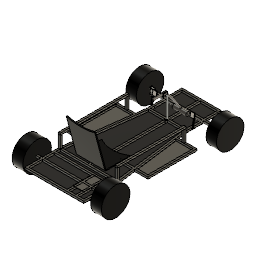
Go Kart Assembly.F3d (Autodesk Fusion 360 archive; units mm, degrees)
design "Go Kart Design"
Autodesk Fusion 360 part; units mm, degrees
note: some values were not read from the file. Chosen so that the rebuilt part matches the saved one: which bodies a step acts on; which face or edge a step refers to. Set by a fixed rule: which sketch regions a step uses.
(part 1 of 2)
sketch "Sketch1" plane through (0, 0, 0) normal (0, 0, 1) x (1, 0, 0)
  line L0 (139.7, 355.6) -> (279.4, 355.6)
  line L1 (279.4, 355.6) -> (279.4, 101.6)
  line L2 (279.4, 101.6) -> (139.7, 101.6)
  line L3 (139.7, 101.6) -> (139.7, 355.6)
  line L4 (139.7, 101.6) -> (160.7997, 101.6)
  line L5 (150.2738, 355.6) -> (139.7, 355.6)
  line L6 (139.7, 355.6) -> (139.7, 101.6)
  line L7 (239.1738, 355.6) -> (279.4, 355.6)
  line L8 (279.4, 355.6) -> (279.4, 101.6)
  line L9 (-508, 228.6) -> (508, 228.6)
  line L10 (508, 228.6) -> (508, 203.2)
  line L11 (508, 203.2) -> (-508, 203.2)
  line L12 (-508, 203.2) -> (-508, 228.6)
  line L13 (139.7, 355.6) -> (165.1, 355.6)
  line L14 (165.1, 355.6) -> (165.1, 25.4)
  line L15 (165.1, 25.4) -> (139.7, 25.4)
  line L16 (139.7, 25.4) -> (139.7, 355.6)
  line L17 (279.4, 355.6) -> (254, 355.6)
  line L18 (254, 355.6) -> (254, 25.4)
  line L19 (254, 25.4) -> (279.4, 25.4)
  line L20 (279.4, 25.4) -> (279.4, 355.6)
  line L21 (381, 457.2) -> (355.6, 457.2)
  line L22 (355.6, 457.2) -> (355.6, 25.4)
  line L23 (355.6, 25.4) -> (381, 25.4)
  line L24 (381, 25.4) -> (381, 457.2)
  line L25 (355.6, 25.4) -> (381, 25.4)
  line L26 (381, 25.4) -> (381, 0)
  line L27 (381, 0) -> (355.6, 0)
  line L28 (355.6, 0) -> (355.6, 25.4)
  line L29 (355.6, 25.4) -> (381, 0)
  line L30 (355.6, 0) -> (-355.6, 0)
  line L31 (-355.6, 0) -> (-355.6, 25.4)
  line L32 (-355.6, 25.4) -> (355.6, 25.4)
  line L33 (355.6, 25.4) -> (355.6, 0)
  line L34 (-355.6, 25.4) -> (-381, 25.4)
  line L35 (-381, 25.4) -> (-381, 0)
  line L36 (-381, 0) -> (-355.6, 0)
  line L37 (-355.6, 0) -> (-355.6, 25.4)
  line L38 (-381, 0) -> (-355.6, 25.4)
  line L39 (-381, 25.4) -> (-355.6, 25.4)
  line L40 (-355.6, 25.4) -> (-355.6, 457.2)
  line L41 (-355.6, 457.2) -> (-381, 457.2)
  line L42 (-381, 457.2) -> (-381, 25.4)
  line L43 (355.6, 355.6) -> (-355.6, 355.6)
  line L44 (-355.6, 355.6) -> (-355.6, 381)
  line L45 (-355.6, 381) -> (355.6, 381)
  line L46 (355.6, 381) -> (355.6, 355.6)
  line L47 (-355.6, 457.2) -> (355.6, 457.2)
  line L48 (355.6, 457.2) -> (355.6, 431.8)
  line L49 (355.6, 431.8) -> (-355.6, 431.8)
  line L50 (-355.6, 431.8) -> (-355.6, 457.2)
  line L51 (254, 1905) -> (-254, 1905)
  line L52 (-254, 1905) -> (244.6512, 1905)
  line L53 (-254, 1879.6) -> (-254, 1905)
  line L54 (-254, 1905) -> (-228.6, 1905)
  line L55 (-228.6, 1905) -> (-228.6, 1701.8)
  line L56 (-228.6, 1701.8) -> (-254, 1701.8)
  line L57 (-254, 1701.8) -> (-254, 1905)
  line L58 (-12.7, 1905) -> (12.7, 1905)
  line L59 (12.7, 1905) -> (12.7, 457.2)
  line L60 (12.7, 457.2) -> (-12.7, 457.2)
  line L61 (-12.7, 457.2) -> (-12.7, 1905)
  line L62 (-254, 1879.6) -> (254, 1879.6)
  line L63 (254, 1905) -> (254, 1879.6)
  line L64 (254, 1905) -> (228.6, 1905)
  line L65 (228.6, 1905) -> (228.6, 1701.8)
  line L66 (228.6, 1701.8) -> (254, 1701.8)
  line L67 (254, 1701.8) -> (254, 1905)
  line L68 (-393.7, 1701.8) -> (393.7, 1701.8)
  line L69 (393.7, 1701.8) -> (393.7, 1676.4)
  line L70 (393.7, 1676.4) -> (-393.7, 1676.4)
  line L71 (-393.7, 1676.4) -> (-393.7, 1701.8)
  line L72 (-254, 1676.4) -> (-228.6, 1676.4)
  line L73 (-228.6, 1676.4) -> (-228.6, 1447.8)
  line L74 (-228.6, 1447.8) -> (-254, 1447.8)
  line L75 (-254, 1447.8) -> (-254, 1676.4)
  line L76 (228.6, 1676.4) -> (254, 1676.4)
  line L77 (254, 1676.4) -> (254, 1447.8)
  line L78 (254, 1447.8) -> (228.6, 1447.8)
  line L79 (228.6, 1447.8) -> (228.6, 1676.4)
  line L80 (-254, 1447.8) -> (-381, 457.2)
  line L81 (254, 1447.8) -> (381, 457.2)
  line L82 (-228.6, 1446.1784) -> (-355.6, 455.5784)
  line L83 (228.6, 1446.1784) -> (355.6, 455.5784)
  line L84 (228.6, 1446.1784) -> (254, 1447.8)
  line L85 (228.6, 1447.8) -> (228.6, 1446.1784)
  line L86 (-254, 1447.8) -> (-228.6, 1446.1784)
  line L87 (-228.6, 1447.8) -> (-228.6, 1446.1784)
  line L88 (-228.6, 1447.8) -> (228.6, 1447.8)
  line L89 (228.6, 1447.8) -> (228.6, 1473.2)
  line L90 (228.6, 1473.2) -> (-228.6, 1473.2)
  line L91 (-228.6, 1473.2) -> (-228.6, 1447.8)
  line L92 (-12.7, 711.2) -> (-322.828, 711.2)
  line L93 (12.7, 711.2) -> (322.828, 711.2)
  line L94 (-12.7, 685.8) -> (-326.0844, 685.8)
  line L95 (12.7, 685.8) -> (326.0844, 685.8)
  line L96 (-270.2821, 1320.8) -> (-524.2821, 1320.8)
  line L97 (270.2821, 1320.8) -> (524.2821, 1320.8)
  line L98 (-524.2821, 1320.8) -> (-524.2821, 685.8)
  line L99 (524.2821, 1320.8) -> (524.2821, 685.8)
  line L100 (-524.2821, 685.8) -> (-351.6923, 685.8)
  line L101 (524.2821, 685.8) -> (351.6923, 685.8)
  line L102 (-498.8821, 1295.4) -> (-273.5385, 1295.4)
  line L103 (-498.8821, 1295.4) -> (-498.8821, 711.2)
  line L104 (-498.8821, 711.2) -> (-348.4359, 711.2)
  line L105 (498.8821, 1295.4) -> (273.5385, 1295.4)
  line L106 (498.8821, 1295.4) -> (498.8821, 711.2)
  line L107 (498.8821, 711.2) -> (348.4359, 711.2)
  line L108 (0, 0) -> (0, 1905)
  point P0 (-12.7, 1905)
  point P1 (-12.7, 685.8)
  point P2 (-270.2821, 1320.8)
  dimension "d20" = 139.7
  dimension "d24" = 25.4
  dimension "d25" = 1016
  dimension "d28" = 101.6
  dimension "d29" = 254
  dimension "d30" = 25.4
  dimension "d31" = 330.2
  dimension "d32" = 25.4
  dimension "d33" = 330.2
  dimension "d35" = 25.4
  dimension "d38" = 76.2
  dimension "d39" = 152.4
  dimension "d41" = 25.4
  dimension "d42" = 25.4
  dimension "d43" = 25.4
  dimension "d44" = 711.2
  dimension "d45" = 25.4
  dimension "d46" = 25.4
  dimension "d47" = 25.4
  dimension "d49" = 177.8
  dimension "d51" = 177.8
  dimension "d56" = 127
  dimension "d57" = 127
  dimension "d58" = 25.4
  dimension "d59" = 711.2
  dimension "d73" = 76.2
  dimension "d74" = 76.2
  dimension "d75" = 25.4
  dimension "d76" = 711.2
  dimension "d118" = 508
  dimension "d119" = 25.4
  dimension "d120" = 25.4
  dimension "d121" = 203.2
  dimension "d125" = 25.4
  dimension "d127" = 508
  dimension "d128" = 203.2
  dimension "d129" = 25.4
  dimension "d130" = 25.4
  dimension "d131" = 787.4
  dimension "d132" = 139.7
  dimension "d133" = 139.7
  dimension "d135" = 25.4
  dimension "d136" = 228.6
  dimension "d137" = 228.6
  dimension "d138" = 25.4
  dimension "d145" = 1905
  dimension "d146" = 25.4
  dimension "d147" = 25.4
  dimension "d148" = 342.9
  dimension "d149" = 342.9
  dimension "d150" = 25.4
  dimension "d151" = 457.2
  dimension "d156" = 254
  dimension "d157" = 254
  dimension "d158" = 25.4
  dimension "d159" = 228.6
  dimension "d160" = 228.6
  dimension "d184" = 254
  dimension "d185" = 254
  dimension "d186" = 635
  dimension "d187" = 635
  dimension "d188" = 172.5897
  dimension "d189" = 172.5897
  dimension "d190" = 25.4
  dimension "d191" = 25.4
  dimension "d192" = 25.4
  dimension "d193" = 25.4
  dimension "d194" = 25.4
  dimension "d195" = 25.4
  dimension "d242" = 1905
  constraint horizontal L0
  constraint vertical L1
  constraint horizontal L2
  constraint vertical L3
  constraint horizontal L5
  constraint vertical L6
  constraint coincident L0 L5.start
  constraint horizontal L7
  constraint vertical L8
  constraint coincident L0 L7.start
  constraint horizontal L9
  constraint vertical L10
  constraint horizontal L11
  constraint vertical L12
  constraint horizontal L13
  constraint vertical L14
  constraint horizontal L15
  constraint vertical L16
  constraint horizontal L17
  constraint vertical L18
  constraint horizontal L19
  constraint vertical L20
  constraint horizontal L21
  constraint vertical L22
  constraint horizontal L23
  constraint vertical L24
  constraint horizontal L25
  constraint vertical L26
  constraint horizontal L27
  constraint vertical L28
  constraint horizontal L30
  constraint vertical L31
  constraint horizontal L32
  constraint vertical L33
  constraint horizontal L34
  constraint vertical L35
  constraint horizontal L36
  constraint vertical L37
  constraint horizontal L39
  constraint vertical L40
  constraint horizontal L41
  constraint vertical L42
  constraint horizontal L43
  constraint vertical L44
  constraint horizontal L45
  constraint vertical L46
  constraint coincident L22 L43.start
  constraint collinear L0 L43
  constraint horizontal L47
  constraint vertical L48
  constraint horizontal L49
  constraint vertical L50
  constraint horizontal L52
  constraint vertical L53
  constraint horizontal L54
  constraint vertical L55
  constraint horizontal L56
  constraint vertical L57
  constraint horizontal L58
  constraint vertical L59
  constraint horizontal L60
  constraint vertical L61
  constraint coincident P0 L58.start
  constraint perpendicular L59 L62
  constraint horizontal L64
  constraint vertical L65
  constraint horizontal L66
  constraint vertical L67
  constraint horizontal L68
  constraint vertical L69
  constraint horizontal L70
  constraint vertical L71
  constraint horizontal L72
  constraint vertical L73
  constraint horizontal L74
  constraint vertical L75
  constraint coincident L70 L72.start
  constraint collinear L57 L75
  constraint horizontal L76
  constraint vertical L77
  constraint horizontal L78
  constraint vertical L79
  constraint coincident L70 L76.start
  constraint collinear L67 L77
  constraint collinear L47 L60
  constraint collinear L51 L58
  constraint parallel L80 L82
  constraint parallel L81 L83
  constraint vertical L85
  constraint vertical L87
  constraint horizontal L88
  constraint vertical L89
  constraint horizontal L90
  constraint vertical L91
  constraint coincident L82 L92.end
  constraint perpendicular L61 L92
  constraint coincident L59 L93.start
  constraint coincident L83 L93.end
  constraint perpendicular L59 L93
  constraint coincident L61 P1
  constraint coincident P1 L94.start
  constraint coincident L82 L94.end
  constraint perpendicular L61 L94
  constraint coincident L59 L95.start
  constraint coincident L83 L95.end
  constraint perpendicular L59 L95
  constraint coincident L80 P2
  constraint coincident P2 L96.start
  constraint horizontal L96
  constraint coincident L81 L97.start
  constraint perpendicular L59 L97
  constraint perpendicular L96 L98
  constraint perpendicular L97 L99
  constraint coincident L80 L100.end
  constraint perpendicular L98 L100
  constraint coincident L81 L101.end
  constraint perpendicular L99 L101
  constraint coincident L80 L102.end
  constraint perpendicular L98 L102
  constraint perpendicular L102 L103
  constraint coincident L80 L104.end
  constraint perpendicular L103 L104
  constraint coincident L81 L105.end
  constraint horizontal L105
  constraint perpendicular L105 L106
  constraint coincident L81 L107.end
  constraint perpendicular L106 L107
  constraint midpoint L108.start L30
  constraint midpoint L58 L108.end
  constraint coincident origin L108
  measures "d20" distance of L0.start L0.end
  measures "d24" distance of L9.start L11.end
  measures "d25" distance of L9.start L9.end
  measures "d28" distance of L2 L11
  measures "d29" distance of L0 L4
  measures "d30" distance of L14 L16
  measures "d31" distance of L13 L15
  measures "d32" distance of L18 L20
  measures "d33" distance of L0 L19
  measures "d35" distance of L21.start L21.end
  measures "d38" distance of L1 L22
  measures "d39" distance of L10 L22
  measures "d41" distance of L26 L28
  measures "d42" distance of L23 L27
  measures "d43" distance of L27.end L22.end
  measures "d44" distance of L27.end L30.end
  measures "d45" distance of L34 L36
  measures "d46" distance of L31 L35
  measures "d47" distance of L40 L42
  measures "d49" distance of L11 L34
  measures "d51" distance of L11 L25
  measures "d56" distance of L12 L42
  measures "d57" distance of L10 L24
  measures "d58" distance of L43.start L45.end
  measures "d59" distance of L44.end L45.end
  measures "d73" distance of L40.end L44.end
  measures "d74" distance of L21.end L45.end
  measures "d75" distance of L40.end L49.end
  measures "d76" distance of L40.end L21.end
  measures "d118" distance of L51.start L51.end
  measures "d119" distance of L51.end L53.start
  measures "d120" distance of L51.end L54.end
  measures "d121" distance of L51.end L56.end
  measures "d125" distance of P0 L58.end
  measures "d127" distance of L53.start L62.end
  measures "d128" distance of L51.start L66.end
  measures "d129" distance of L65.end L66.end
  measures "d130" distance of L68.start L70.end
  measures "d131" distance of L68.start L68.end
  measures "d132" distance of L56.end L68.start
  measures "d133" distance of L66.end L68.end
  measures "d135" distance of L73.end L74.end
  measures "d136" distance of L72.end L73.end
  measures "d137" distance of L76.start L78.end
  measures "d138" distance of L77.end L78.end
  measures "d145" distance of L30 L52
  measures "d146" distance of L80 L82
  measures "d147" distance of L81 L83
  measures "d148" distance of L40.end L60.end
  measures "d149" horizontal distance of L59.end L83.end
  measures "d150" distance of L73.end L90.end
  measures "d151" distance of L89.end L90.end
  measures "d156" distance of L47 L92
  measures "d157" distance of L47 L93
  measures "d158" distance of L92.start P1
  measures "d159" distance of L47 L95
  measures "d160" distance of L47 L94
  measures "d184" distance of P2 L96.end
  measures "d185" distance of L97.start L97.end
  measures "d186" distance of L96.end L98.end
  measures "d187" distance of L97.end L99.end
  measures "d188" distance of L98.end L100.end
  measures "d189" distance of L99.end L101.end
  measures "d190" distance of L96 L102
  measures "d191" distance of L98 L102.start
  measures "d192" distance of L100 L103.end
  measures "d193" distance of L97 L105
  measures "d194" distance of L99 L105.start
  measures "d195" distance of L101 L106.end
  measures "d242" distance of L108.start L108.end
extrude "Extrude1" add sketch "Sketch1" along normal blind 25.4 contours L0 L5 L7 L13 L17 L22 L43 L45 L46 L108 | L0 L3 L5 L6 L9 L13 L14 L16 L43 | L3 L6 L9 L11 L14 L16 | L3 L6 L9 L11 L16 L108 | L40 L43 L44 L45 L108 | L2 L3 L4 L6 L11 L14 L16 | L9 L11 L40 L108 | L9 L11 L14 L18 | L9 L40 L41 L42 L44 L50 | L2 L4 L14 L15 L16 L32 | L9 L11 L40 L42 | L0 L1 L7 L8 L9 L17 L18 L20 L43 | L1 L8 L9 L11 L18 L20 | L9 L21 L22 L24 L46 L48 | L22 L47 L48 L49 L60 L83 L108 | L40 L47 L49 L50 L60 L82 L108 | L15 L19 L28 L30 L32 L33 L108 | L1 L2 L8 L11 L18 L20 | L11 L34 L39 L40 L42 | L30 L31 L32 L37 L108 | L9 L11 L12 L42 | L1 L8 L9 L11 L20 L22 | L47 L59 L60 L88 L108 | L47 L60 L61 L88 L108 | L2 L18 L19 L20 L32 | L34 L35 L38 L39 | L31 L36 L37 L38 | L41 L47 L80 L82 L86 | L9 L11 L22 L24 | L59 L88 L90 L108 | L61 L88 L90 L108 | L11 L22 L23 L24 L25 | L27 L28 L29 L33 | L9 L10 L11 L24 | L21 L47 L81 L83 L84 | L61 L82 L92 L94 | L59 L83 L93 L95 | L61 L73 L88 L90 L91 | L59 L79 L88 L89 L90 | L59 L70 L90 L108 | L61 L70 L90 L108 | L23 L25 L26 L29 | L70 L72 L73 L74 L75 L91 | L74 L86 L87 | L70 L76 L77 L78 L79 L89 | L78 L84 L85 | L59 L68 L70 L108 | L61 L68 L70 L108 | L56 L61 L68 L70 L71 L72 | L59 L66 L68 L69 L70 L76 | L59 L62 L68 L108 | L61 L62 L68 L108 | L51 L52 L58 L59 L62 L108 | L51 L52 L58 L61 L62 L108 | L51 L52 L55 L61 L62 | L55 L56 L57 L62 L68 | L51 L52 L59 L62 L65 | L62 L65 L66 L67 L68 | L51 L52 L53 L54 L55 L57 L62 | L51 L52 L62 L63 L64 L65 L67 makes body 1
sketch "Sketch3" plane through (0, 0, 0) normal (0, 0, -1) x (1, 0, 0)
  line L0 (355.6, -203.2) -> (279.4, -203.2)
  line L1 (279.4, -203.2) -> (279.4, -25.4)
  line L2 (279.4, -25.4) -> (355.6, -25.4)
  line L3 (355.6, -25.4) -> (355.6, -203.2)
  line L4 (228.6, -1879.6) -> (12.7, -1879.6)
  line L5 (12.7, -1879.6) -> (12.7, -1701.8)
  line L6 (12.7, -1701.8) -> (228.6, -1701.8)
  line L7 (228.6, -1701.8) -> (228.6, -1879.6)
  line L8 (-12.7, -1473.2) -> (-12.7, -1676.4)
  line L9 (-12.7, -1676.4) -> (-228.6, -1676.4)
  line L10 (-228.6, -1676.4) -> (-228.6, -1473.2)
  line L11 (-228.6, -1473.2) -> (-12.7, -1473.2)
  line L12 (355.3921, -457.2) -> (355.6, -455.5784)
  line L13 (355.6, -455.5784) -> (355.6, -457.2)
  line L14 (355.6, -457.2) -> (355.3921, -457.2)
  line L15 (355.3921, -457.2) -> (326.0844, -685.8)
  line L16 (326.0844, -685.8) -> (12.7, -685.8)
  line L17 (12.7, -685.8) -> (12.7, -457.2)
  line L18 (12.7, -457.2) -> (355.3921, -457.2)
  line L19 (228.6, -1676.4) -> (12.7, -1676.4)
  line L20 (12.7, -1676.4) -> (12.7, -1473.2)
  line L21 (12.7, -1473.2) -> (228.6, -1473.2)
  line L22 (228.6, -1473.2) -> (228.6, -1676.4)
  line L23 (279.4, -228.6) -> (355.6, -228.6)
  line L24 (355.6, -228.6) -> (355.6, -355.6)
  line L25 (355.6, -355.6) -> (279.4, -355.6)
  line L26 (279.4, -355.6) -> (279.4, -228.6)
  line L27 (12.7, -1447.8) -> (12.7, -711.2)
  line L28 (12.7, -711.2) -> (322.828, -711.2)
  line L29 (322.828, -711.2) -> (228.6, -1446.1784)
  line L30 (228.6, -1446.1784) -> (228.6, -1447.8)
  line L31 (228.6, -1447.8) -> (12.7, -1447.8)
  line L32 (-228.6, -1879.6) -> (-228.6, -1701.8)
  line L33 (-228.6, -1701.8) -> (-12.7, -1701.8)
  line L34 (-12.7, -1701.8) -> (-12.7, -1879.6)
  line L35 (-12.7, -1879.6) -> (-228.6, -1879.6)
  line L36 (254, -203.2) -> (165.1, -203.2)
  line L37 (165.1, -203.2) -> (165.1, -25.4)
  line L38 (165.1, -25.4) -> (254, -25.4)
  line L39 (254, -25.4) -> (254, -203.2)
  line L40 (139.7, -25.4) -> (139.7, -203.2)
  line L41 (139.7, -203.2) -> (-355.6, -203.2)
  line L42 (-355.6, -203.2) -> (-355.6, -25.4)
  line L43 (-355.6, -25.4) -> (139.7, -25.4)
  line L44 (254, -355.6) -> (165.1, -355.6)
  line L45 (165.1, -355.6) -> (165.1, -228.6)
  line L46 (165.1, -228.6) -> (254, -228.6)
  line L47 (254, -228.6) -> (254, -355.6)
  line L48 (-228.6, -1447.8) -> (-228.6, -1446.1784)
  line L49 (-228.6, -1446.1784) -> (-322.828, -711.2)
  line L50 (-322.828, -711.2) -> (-12.7, -711.2)
  line L51 (-12.7, -711.2) -> (-12.7, -1447.8)
  line L52 (-12.7, -1447.8) -> (-228.6, -1447.8)
  line L53 (-12.7, -457.2) -> (-12.7, -685.8)
  line L54 (-12.7, -685.8) -> (-326.0844, -685.8)
  line L55 (-326.0844, -685.8) -> (-355.3921, -457.2)
  line L56 (-355.3921, -457.2) -> (-355.6, -457.2)
  line L57 (-355.6, -457.2) -> (-355.6, -455.5784)
  line L58 (-355.6, -455.5784) -> (-355.3921, -457.2)
  line L59 (-355.3921, -457.2) -> (-12.7, -457.2)
  line L60 (-355.6, -381) -> (355.6, -381)
  line L61 (355.6, -381) -> (355.6, -431.8)
  line L62 (355.6, -431.8) -> (-355.6, -431.8)
  line L63 (-355.6, -431.8) -> (-355.6, -381)
  line L64 (-355.6, -228.6) -> (139.7, -228.6)
  line L65 (139.7, -228.6) -> (139.7, -355.6)
  line L66 (139.7, -355.6) -> (-355.6, -355.6)
  line L67 (-355.6, -355.6) -> (-355.6, -228.6)
  line L68 (254, -1905) -> (254, -1701.8)
  line L69 (254, -1701.8) -> (393.7, -1701.8)
  line L70 (393.7, -1701.8) -> (393.7, -1676.4)
  line L71 (393.7, -1676.4) -> (254, -1676.4)
  line L72 (254, -1676.4) -> (254, -1447.8)
  line L73 (254, -1447.8) -> (381, -457.2)
  line L74 (381, -457.2) -> (381, -228.6)
  line L75 (381, -228.6) -> (508, -228.6)
  line L76 (508, -228.6) -> (508, -203.2)
  line L77 (508, -203.2) -> (381, -203.2)
  line L78 (381, -203.2) -> (381, 0)
  line L79 (381, 0) -> (-381, 0)
  line L80 (-381, 0) -> (-381, -203.2)
  line L81 (-381, -203.2) -> (-508, -203.2)
  line L82 (-508, -203.2) -> (-508, -228.6)
  line L83 (-508, -228.6) -> (-381, -228.6)
  line L84 (-381, -228.6) -> (-381, -457.2)
  line L85 (-381, -457.2) -> (-254, -1447.8)
  line L86 (-254, -1447.8) -> (-254, -1676.4)
  line L87 (-254, -1676.4) -> (-393.7, -1676.4)
  line L88 (-393.7, -1676.4) -> (-393.7, -1701.8)
  line L89 (-393.7, -1701.8) -> (-254, -1701.8)
  line L90 (-254, -1701.8) -> (-254, -1905)
  line L91 (-254, -1905) -> (254, -1905)
  line L92 (254, -1905) -> (-254, -1905)
  line L93 (-254, -1447.8) -> (-381, -457.2)
  line L94 (-254, -1905) -> (-254, -1447.8)
  line L95 (-381, -457.2) -> (-381, 0)
  line L96 (381, 0) -> (-381, 0)
  line L97 (381, -457.2) -> (381, 0)
  line L98 (381, -457.2) -> (254, -1447.8)
  line L99 (254, -1447.8) -> (254, -1905)
  constraint coincident L68.start L91.end
  constraint coincident L90.end L91.start
  constraint coincident L85.end L86.start
  constraint coincident L84.end L85.start
  constraint coincident L79.end L80.start
  constraint coincident L78.end L79.start
  constraint coincident L73.end L74.start
  constraint coincident L72.end L73.start
extrude "Extrude2" add sketch "Sketch3" along normal blind 1.6002 separate body contours L0 L1 L2 L3 | L4 L5 L6 L7 | L8 L9 L10 L11 | L15 L16 L17 L18 | L19 L20 L21 L22 | L23 L24 L25 L26 | L27 L28 L29 L30 L31 | L32 L33 L34 L35 | L36 L37 L38 L39 | L40 L41 L42 L43 | L44 L45 L46 L47 | L48 L49 L50 L51 L52 | L53 L54 L55 L59 | L60 L61 L62 L63 | L64 L65 L66 L67 | L68 L72 L73 L74 L78 L79 L80 L84 L85 L86 L90 L91 L92 L93 L94 L95 L96 L97 L98 L99 makes body 2
sketch "Sketch4" plane through (0, 0, 25.4) normal (0, 0, 1) x (-1, 0, 0)
  line L0 (-279.4, -203.2) -> (-355.6, -203.2)
  line L1 (-355.6, -203.2) -> (-355.6, -25.4)
  line L2 (-355.6, -25.4) -> (-279.4, -25.4)
  line L3 (-279.4, -25.4) -> (-279.4, -203.2)
  line L4 (-12.7, -1879.6) -> (-228.6, -1879.6)
  line L5 (-228.6, -1879.6) -> (-228.6, -1701.8)
  line L6 (-228.6, -1701.8) -> (-12.7, -1701.8)
  line L7 (-12.7, -1701.8) -> (-12.7, -1879.6)
  line L8 (12.7, -1676.4) -> (12.7, -1473.2)
  line L9 (12.7, -1473.2) -> (228.6, -1473.2)
  line L10 (228.6, -1473.2) -> (228.6, -1676.4)
  line L11 (228.6, -1676.4) -> (12.7, -1676.4)
  line L12 (-355.6, -455.5784) -> (-355.3921, -457.2)
  line L13 (-355.3921, -457.2) -> (-12.7, -457.2)
  line L14 (-12.7, -457.2) -> (-12.7, -685.8)
  line L15 (-12.7, -685.8) -> (-326.0844, -685.8)
  line L16 (-326.0844, -685.8) -> (-355.3921, -457.2)
  line L17 (-355.3921, -457.2) -> (-355.6, -457.2)
  line L18 (-355.6, -457.2) -> (-355.6, -455.5784)
  line L19 (-12.7, -1676.4) -> (-228.6, -1676.4)
  line L20 (-228.6, -1676.4) -> (-228.6, -1473.2)
  line L21 (-228.6, -1473.2) -> (-12.7, -1473.2)
  line L22 (-12.7, -1473.2) -> (-12.7, -1676.4)
  line L23 (-355.6, -228.6) -> (-279.4, -228.6)
  line L24 (-279.4, -228.6) -> (-279.4, -355.6)
  line L25 (-279.4, -355.6) -> (-355.6, -355.6)
  line L26 (-355.6, -355.6) -> (-355.6, -228.6)
  line L27 (-12.7, -711.2) -> (-12.7, -1447.8)
  line L28 (-12.7, -1447.8) -> (-228.6, -1447.8)
  line L29 (-228.6, -1447.8) -> (-228.6, -1446.1784)
  line L30 (-228.6, -1446.1784) -> (-322.828, -711.2)
  line L31 (-322.828, -711.2) -> (-12.7, -711.2)
  line L32 (228.6, -1701.8) -> (228.6, -1879.6)
  line L33 (228.6, -1879.6) -> (12.7, -1879.6)
  line L34 (12.7, -1879.6) -> (12.7, -1701.8)
  line L35 (12.7, -1701.8) -> (228.6, -1701.8)
  line L36 (-165.1, -203.2) -> (-254, -203.2)
  line L37 (-254, -203.2) -> (-254, -25.4)
  line L38 (-254, -25.4) -> (-165.1, -25.4)
  line L39 (-165.1, -25.4) -> (-165.1, -203.2)
  line L40 (-139.7, -203.2) -> (-139.7, -25.4)
  line L41 (-139.7, -25.4) -> (355.6, -25.4)
  line L42 (355.6, -25.4) -> (355.6, -203.2)
  line L43 (355.6, -203.2) -> (-139.7, -203.2)
  line L44 (-165.1, -355.6) -> (-254, -355.6)
  line L45 (-254, -355.6) -> (-254, -228.6)
  line L46 (-254, -228.6) -> (-165.1, -228.6)
  line L47 (-165.1, -228.6) -> (-165.1, -355.6)
  line L48 (228.6, -1446.1784) -> (228.6, -1447.8)
  line L49 (228.6, -1447.8) -> (12.7, -1447.8)
  line L50 (12.7, -1447.8) -> (12.7, -711.2)
  line L51 (12.7, -711.2) -> (322.828, -711.2)
  line L52 (322.828, -711.2) -> (228.6, -1446.1784)
  line L53 (12.7, -685.8) -> (12.7, -457.2)
  line L54 (12.7, -457.2) -> (355.3921, -457.2)
  line L55 (355.3921, -457.2) -> (355.6, -455.5784)
  line L56 (355.6, -455.5784) -> (355.6, -457.2)
  line L57 (355.6, -457.2) -> (355.3921, -457.2)
  line L58 (355.3921, -457.2) -> (326.0844, -685.8)
  line L59 (326.0844, -685.8) -> (12.7, -685.8)
  line L60 (-355.6, -381) -> (355.6, -381)
  line L61 (355.6, -381) -> (355.6, -431.8)
  line L62 (355.6, -431.8) -> (-355.6, -431.8)
  line L63 (-355.6, -431.8) -> (-355.6, -381)
  line L64 (-139.7, -228.6) -> (355.6, -228.6)
  line L65 (355.6, -228.6) -> (355.6, -355.6)
  line L66 (355.6, -355.6) -> (-139.7, -355.6)
  line L67 (-139.7, -355.6) -> (-139.7, -228.6)
  line L68 (-254, -1701.8) -> (-254, -1905)
  line L69 (-254, -1905) -> (254, -1905)
  line L70 (254, -1905) -> (254, -1701.8)
  line L71 (254, -1701.8) -> (393.7, -1701.8)
  line L72 (393.7, -1701.8) -> (393.7, -1676.4)
  line L73 (393.7, -1676.4) -> (254, -1676.4)
  line L74 (254, -1676.4) -> (254, -1447.8)
  line L75 (254, -1447.8) -> (381, -457.2)
  line L76 (381, -457.2) -> (381, -228.6)
  line L77 (381, -228.6) -> (508, -228.6)
  line L78 (508, -228.6) -> (508, -203.2)
  line L79 (508, -203.2) -> (381, -203.2)
  line L80 (381, -203.2) -> (381, 0)
  line L81 (381, 0) -> (-381, 0)
  line L82 (-381, 0) -> (-381, -203.2)
  line L83 (-381, -203.2) -> (-508, -203.2)
  line L84 (-508, -203.2) -> (-508, -228.6)
  line L85 (-508, -228.6) -> (-381, -228.6)
  line L86 (-381, -228.6) -> (-381, -457.2)
  line L87 (-381, -457.2) -> (-254, -1447.8)
  line L88 (-254, -1447.8) -> (-254, -1676.4)
  line L89 (-254, -1676.4) -> (-393.7, -1676.4)
  line L90 (-393.7, -1676.4) -> (-393.7, -1701.8)
  line L91 (-393.7, -1701.8) -> (-254, -1701.8)
  line L92 (-139.7, -355.6) -> (-139.7, -101.6)
  line L93 (-279.4, -355.6) -> (-279.4, -101.6)
  line L94 (-139.7, -101.6) -> (-279.4, -101.6)
  line L95 (-139.7, -355.6) -> (-279.4, -355.6)
  dimension "d179" = 254
  dimension "d180" = 254
  constraint coincident L66.end L67.start
  constraint perpendicular L64 L92
  constraint coincident L24.end L25.start
  constraint perpendicular L23 L93
  measures "d179" distance of L66.end L92.end
  measures "d180" distance of L24.end L93.end
extrude "Extrude3" add sketch "Sketch4" along normal blind 3.8 separate body contours L3 L24 L36 L37 L39 L40 L45 L46 L47 L67 L92 L93 L94 L95 | L36 L37 L39 L94 | L44 L45 L46 L47 L95 makes body 3
ref_plane "WorkPlane1" through (184.0461, 457.2, 25.4) normal (0, 0.965926, 0.258819) x (-1, 0, 0)
extrude "Extrude5" add sketch "Sketch1" along normal blind 25.4 separate body contours L80 L96 L98 L100 L102 L103 L104 | L81 L97 L99 L101 L105 L106 L107 makes body 4 at (-515.8154, 905.9333, 0) makes body 5 at (515.8154, 905.9333, 0)
extrude "Extrude6" add sketch "Sketch1" along normal blind 1.6002 contours L80 L102 L103 L104 | L81 L105 L106 L107 bodies 1 3 4 2 5
sketch "Sketch10" plane through (-393.7, 0, 0) normal (-1, 0, 0) x (0, -1, 0)
  line L0 (-1701.8, 0) -> (-1676.4, 0)
  line L1 (-1676.4, 0) -> (-1676.4, 25.4)
  line L2 (-1676.4, 25.4) -> (-1701.8, 25.4)
  line L3 (-1701.8, 25.4) -> (-1701.8, 0)
  line L4 (-1701.8, 50.8) -> (-1701.8, -25.4)
  line L5 (-1701.8, 50.8) -> (-1676.4, 50.8)
  line L6 (-1676.4, 50.8) -> (-1676.4, -25.4)
  line L7 (-1676.4, -25.4) -> (-1701.8, -25.4)
  line L8 (-1701.8, -25.4) -> (-1701.8, 50.8)
  line L9 (-1701.8, 44.45) -> (-1676.4, 44.45)
  line L10 (-1701.8, -19.05) -> (-1676.4, -19.05)
  point P0 (-1701.8, 12.7)
  point P1 (-1701.8, 12.7)
  dimension "d215" = 25.4
  dimension "d216" = 12.7
  dimension "d217" = 76.2
  dimension "d218" = 76.2
  dimension "d219" = 6.35
  dimension "d220" = 6.35
  constraint coincident L3 P1
  constraint midpoint L4 P1
  constraint coincident P1 P0
  constraint parallel L3 L4
  constraint horizontal L5
  constraint vertical L6
  constraint horizontal L7
  constraint vertical L8
  constraint coincident L4 L9.start
  constraint coincident L6 L9.end
  constraint perpendicular L6 L9
  constraint coincident L4 L10.start
  constraint coincident L6 L10.end
  constraint perpendicular L6 L10
  measures "d215" distance of L1 P1
  measures "d216" distance of L0.start P0
  measures "d217" distance of L4.start L4.end
  measures "d218" distance of L4.start L4.end
  measures "d219" distance of L5 L9
  measures "d220" distance of L7 L10
extrude "Extrude9" add sketch "Sketch10" along normal blind 50.8 separate body contours L4 L6 L7 L8 L10 | L4 L5 L6 L8 L9 makes body 6 at (-427.5667, 1693.3333, 50.8) makes body 7 at (-427.5667, 1693.3333, -19.05)
extrude "Extrude10" add sketch "Sketch10" along normal blind 6.35 contours L0 L1 L2 L3 L4 L6 L8 | L0 L4 L6 L8 L10 | L2 L4 L6 L8 L9 bodies 1 3 6 7
sketch "Sketch11" plane through (0, 0, 50.8) normal (0, 0, 1) x (-1, 0, 0)
  line L0 (393.7, -1676.4) -> (393.7, -1701.8)
  line L1 (393.7, -1701.8) -> (444.5, -1701.8)
  line L2 (444.5, -1701.8) -> (444.5, -1676.4)
  line L3 (444.5, -1676.4) -> (393.7, -1676.4)
  circle A0 centre (430.2125, -1689.1) radius 7.9375
  line L4 (422.275, -1697.0375) -> (438.15, -1697.0375)
  line L5 (422.275, -1681.1625) -> (438.15, -1681.1625)
  line L6 (438.15, -1681.1625) -> (422.275, -1681.1625)
  line L7 (422.275, -1681.1625) -> (422.275, -1680.1625)
  line L8 (422.275, -1680.1625) -> (438.15, -1680.1625)
  line L9 (438.15, -1680.1625) -> (438.15, -1681.1625)
  line L10 (438.15, -1697.0375) -> (422.275, -1697.0375)
  line L11 (422.275, -1697.0375) -> (422.275, -1698.0375)
  line L12 (422.275, -1698.0375) -> (438.15, -1698.0375)
  line L13 (438.15, -1698.0375) -> (438.15, -1697.0375)
  point P0 (430.2125, -1689.1)
  point P1 (430.2125, -1697.0375)
  point P2 (430.2125, -1681.1625)
  point P3 (430.2125, -1697.0375)
  point P4 (430.2125, -1681.1625)
  dimension "d225" = 12.7
  dimension "d226" = 14.2875
  dimension "d227" = 15.875
  dimension "d233" = 15.875
  dimension "d234" = 15.875
  dimension "d235" = 1
  dimension "d236" = 1
  constraint coincident P0 A0.centre
  constraint coincident A0 P3
  constraint coincident A0 P4
  constraint midpoint L4 P3
  constraint coincident P3 P1
  constraint horizontal L4
  constraint midpoint L5 P4
  constraint coincident P4 P2
  constraint horizontal L5
  constraint horizontal L6
  constraint vertical L7
  constraint horizontal L8
  constraint vertical L9
  constraint horizontal L10
  constraint vertical L11
  constraint horizontal L12
  constraint vertical L13
  measures "d225" distance of L3 P0
  measures "d226" distance of L2 P0
  measures "d227" diameter of A0
  measures "d233" distance of L4.start L4.end
  measures "d234" distance of L5.start L5.end
  measures "d235" distance of L5.end L8.end
  measures "d236" distance of L4.end L12.end
extrude "Extrude11" add sketch "Sketch11" along normal blind 12.7 and the other way blind 101.6 separate body contours A0 makes body 8
sketch "Sketch13" plane through (-438.15, 0, 0) normal (-1, 0, 0) x (0, -1, 0)
  line L0 (-1697.0375, -50.8) -> (-1697.0375, 63.5)
  line L1 (-1697.0375, 63.5) -> (-1698.0375, 63.5)
  line L2 (-1698.0375, 63.5) -> (-1698.0375, -50.8)
  line L3 (-1698.0375, -50.8) -> (-1697.0375, -50.8)
  circle A0 centre (-1689.1, 30) radius 7.9375
  dimension "d237" = 15.875
  dimension "d238" = 8.9375
  measures "d237" diameter of A0
  measures "d238" distance of L2 A0.centre
extrude "Extrude12" add sketch "Sketch13" along normal blind 114.3 separate body contours A0 makes body 9
split "Split1" by plane through (-393.7, 0, 0) normal (1, 0, 0) bodies 1 makes body 10 at (-469.9, 228.6, 8.4667) makes body 11 at (-480.7547, 897.4667, 0) makes body 12 at (-84.6667, 787.4, -1.6002)
mirror "Mirror1" about plane through (0, 0, 0) normal (1, 0, 0) of bodies 1 8 9 makes body 13 at (400.05, 1693.3333, 23.2833) makes body 14 at (425.1104, 1683.0195, -16.9333) makes body 15 at (476.25, 1691.2498, 37.6408)
combine "Combine1" operation add target body 12 tool bodies 11
split "Split2" by plane through (0, 0, 0) normal (0, 0, 1) bodies 12 makes body 16 at (46.5667, 8.4667, 25.4)
sketch "Sketch16" plane through (-393.7, 0, 0) normal (1, 0, 0) x (0, 1, 0)
  line L0 (1701.8, -25.4) -> (1701.8, 50.8)
  line L1 (1701.8, 50.8) -> (1676.4, 50.8)
  line L2 (1676.4, 50.8) -> (1676.4, -25.4)
  line L3 (1676.4, -25.4) -> (1701.8, -25.4)
  line L4 (1701.8, 25.4) -> (1676.4, 25.4)
  circle A0 centre (1638.3, 38.1) radius 4.7625
  circle A1 centre (1638.3, 38.1) radius 25.4
  point P0 (1676.4, 38.1)
  point P1 (1638.3, 38.1)
  dimension "d246" = 12.7
  dimension "d247" = 38.1
  dimension "d248" = 9.525
  dimension "d249" = 50.8
  constraint coincident L2 P0
  constraint coincident P1 A0.centre
  constraint concentric A0 A1
  measures "d246" distance of P0 L4
  measures "d247" distance of P0 P1
  measures "d248" diameter of A0
  measures "d249" diameter of A1
extrude "Extrude13" add sketch "Sketch16" along normal blind 787.4 separate body contours A0 makes body 17
extrude "Extrude14" add sketch "Sketch16" along normal blind 177.8 from surface at 304.8 separate body contours A1 makes body 18
ref_plane "WorkPlane3" through (-120.65, 1676.4, 25.4) normal (0, -0.819152, -0.573576) x (1, 0, 0)
sketch "Sketch18" plane through (0, 1136.8154, 796.0067) normal (0, -0.819152, -0.573576) x (1, 0, 0)
  line L0 (-12.7169, -880.4638) -> (12.6831, -880.4638)
  line L1 (12.6831, -880.4638) -> (12.6831, -537.5638)
  line L2 (12.6831, -537.5638) -> (-12.7169, -537.5638)
  line L3 (-12.7169, -537.5638) -> (-12.7169, -880.4638)
  dimension "d256" = 25.4
  dimension "d257" = 342.9
  dimension "d258" = 25.4
  constraint horizontal L0
  constraint perpendicular L0 L1
  constraint perpendicular L1 L2
  measures "d256" distance of L0.start L0.end
  measures "d257" distance of L0.end L1.end
  measures "d258" distance of L1.end L2.end
extrude "Extrude15" add sketch "Sketch18" along normal blind 25.4 separate body makes body 19
sketch "Sketch19" plane through (0, 308.3339, -440.3465) normal (0, -0.573576, 0.819152) x (1, 0, 0)
  line L0 (12.6831, 1387.7953) -> (-12.7169, 1387.7953)
  line L1 (-12.7169, 1387.7953) -> (-12.7169, 1362.3953)
  line L2 (-12.7169, 1362.3953) -> (12.6831, 1362.3953)
  line L3 (12.6831, 1362.3953) -> (12.6831, 1387.7953)
  line L4 (-12.7169, 1387.7953) -> (-122.7021, 1451.2953)
  line L5 (12.6831, 1387.7953) -> (122.6683, 1451.2953)
  line L6 (-12.7169, 1387.7953) -> (12.6831, 1387.7953)
  line L7 (-122.7021, 1451.2953) -> (-148.1021, 1407.3012)
  line L8 (-148.1021, 1407.3012) -> (-139.2808, 1357.273)
  line L9 (-139.2808, 1357.273) -> (-109.7227, 1315.9576)
  line L10 (-109.7227, 1315.9576) -> (-12.7169, 1362.3953)
  line L11 (-12.7169, 1362.3953) -> (12.6831, 1362.3953)
  line L12 (122.6683, 1451.2953) -> (148.0683, 1407.3012)
  line L13 (148.0683, 1407.3012) -> (139.247, 1357.273)
  line L14 (139.247, 1357.273) -> (109.6751, 1315.9675)
  line L15 (12.6831, 1362.3953) -> (109.6751, 1315.9675)
  dimension "d262" = 127
  dimension "d263" = 120
  dimension "d264" = 127
  dimension "d265" = 120
  dimension "d266" = 50.8
  dimension "d269" = 50.8
  dimension "d270" = 50.8
  dimension "d271" = 140
  dimension "d272" = 100
  dimension "d273" = 50.8
  dimension "d274" = 90
  dimension "d275" = 50.8
  dimension "d276" = 140
  dimension "d277" = 50.8
  dimension "d278" = 154.4
  constraint coincident L0.end L1.start
  constraint coincident L0.start L3.end
  constraint perpendicular L4 L7
  constraint coincident L1.end L2.start
  constraint coincident L2.end L3.start
  measures "d262" distance of L0.end L4.end
  measures "d263" angle of L1 L4
  measures "d264" distance of L0.start L5.end
  measures "d265" angle of L3 L5
  measures "d266" distance of L4.end L7.end
  measures "d269" distance of L7.end L8.end
  measures "d270" distance of L8.end L9.end
  measures "d271" angle of L7 L8
  measures "d272" angle of L9 L10
  measures "d273" distance of L5.end L12.end
  measures "d274" angle of L5 L12
  measures "d275" distance of L12.end L13.end
  measures "d276" angle of L12 L13
  measures "d277" distance of L13.end L14.end
  measures "d278" angle of L13 L14
extrude "Extrude16" add sketch "Sketch19" along normal blind 25.4 bodies 19
sketch "Sketch20" plane through (-254, 0, 0) normal (-1, 0, 0) x (0, -1, 0)
  line L0 (-1676.4, 0) -> (-1447.8, 0)
  line L1 (-1447.8, 0) -> (-1447.8, 25.4)
  line L2 (-1447.8, 25.4) -> (-1676.4, 25.4)
  line L3 (-1676.4, 25.4) -> (-1676.4, 0)
  circle A0 centre (-1524, 12.78) radius 5
  point P0 (-1524, 12.78)
  dimension "d282" = 12.78
  dimension "d283" = 152.4
  dimension "d284" = 10
  constraint coincident P0 A0.centre
  measures "d282" distance of L0 P0
  measures "d283" distance of L3 P0
  measures "d284" diameter of A0
extrude "Extrude17" cut sketch "Sketch20" against normal blind 25.4 contours A0 bodies 16
extrude "Extrude18" cut sketch "Sketch20" against normal blind 25.4 from surface at -482.6 contours A0 bodies 16
extrude "Extrude19" add sketch "Sketch20" along normal blind 12.7 and the other way blind 38.1 separate body contours A0 makes body 20
extrude "Extrude20" add sketch "Sketch20" against normal blind 50.8 from surface at -469.9 separate body contours A0 makes body 21
sketch "Sketch21" plane through (-266.7, 0, 0) normal (-1, 0, 0) x (0, -1, 0)
  circle A0 centre (-1524, 12.78) radius 5
  line L0 (-1528.9242, 11.9124) -> (-1557.5529, 174.4098)
  line L1 (-1519.0758, 13.6475) -> (-1547.7046, 176.1449)
  line L2 (-1547.663, 118.2743) -> (-1537.8147, 120.0094)
  line L3 (-1557.5529, 174.4098) -> (-1547.7046, 176.1449)
  arc A1 (-1528.9242, 11.9124) -> (-1519.0758, 13.6475) centre (-1524, 12.78) ccw
  circle A2 centre (-1528.4371, 37.965) radius 3
  circle A3 centre (-1530.1989, 47.965) radius 3
  circle A4 centre (-1531.9607, 57.965) radius 3
  circle A5 centre (-1533.7225, 67.965) radius 3
  dimension "d297" = 165
  dimension "d298" = 165
  dimension "d299" = 57
  dimension "d300" = 6
  dimension "d301" = 10
  dimension "d302" = 5
  dimension "d304" = 6
  dimension "d305" = 6
  dimension "d306" = 6
  dimension "d307" = 5
  dimension "d308" = 5
  dimension "d309" = 5
  dimension "d310" = 10
  dimension "d311" = 10
  dimension "d312" = 10
  dimension "d313" = 25.185
  constraint coincident A0 L0.start
  constraint coincident A0 L1.start
  constraint parallel L0 L1
  constraint coincident L0 L2.start
  constraint coincident L1 L2.end
  constraint perpendicular L1 L2
  constraint parallel L2 L3
  measures "d297" distance of L0.start L0.end
  measures "d298" distance of L1.start L1.end
  measures "d299" distance of L2 L3
  measures "d300" diameter of A2
  measures "d301" distance of L0 L1
  measures "d302" distance of L0 A2.centre
  measures "d304" diameter of A3
  measures "d305" diameter of A4
  measures "d306" diameter of A5
  measures "d307" distance of L0 A5.centre
  measures "d308" distance of L0 A4.centre
  measures "d309" distance of L0 A3.centre
  measures "d310" vertical distance of A2.centre A3.centre
  measures "d311" vertical distance of A3.centre A4.centre
  measures "d312" vertical distance of A4.centre A5.centre
  measures "d313" vertical distance of A0.centre A2.centre
extrude "Extrude21" add sketch "Sketch21" along normal blind 6.35 bodies 20
extrude "Extrude22" add sketch "Sketch21" against normal blind 44 contours L0 L1 L2 L3 bodies 20
extrude "Extrude23" add sketch "Sketch21" along normal blind 6.35 from surface at -533.4 bodies 21
extrude "Extrude24" add sketch "Sketch21" along normal blind 50.35 from surface at -533.4 contours L0 L1 L2 L3 bodies 21
sketch "Sketch22" plane through (0, 0, 25.4) normal (0, 0, 1) x (-1, 0, 0)
  line L0 (498.8821, -1295.4) -> (273.5385, -1295.4)
  line L1 (273.5385, -1295.4) -> (348.4359, -711.2)
  line L2 (348.4359, -711.2) -> (498.8821, -711.2)
  line L3 (498.8821, -711.2) -> (498.8821, -1295.4)
  line L4 (-12.7, -1879.6) -> (-228.6, -1879.6)
  line L5 (-228.6, -1879.6) -> (-228.6, -1701.8)
  line L6 (-228.6, -1701.8) -> (-12.7, -1701.8)
  line L7 (-12.7, -1701.8) -> (-12.7, -1879.6)
  line L8 (-279.4, -203.2) -> (-355.6, -203.2)
  line L9 (-355.6, -203.2) -> (-355.6, -25.4)
  line L10 (-355.6, -25.4) -> (-279.4, -25.4)
  line L11 (-279.4, -25.4) -> (-279.4, -203.2)
  line L12 (12.7, -1676.4) -> (12.7, -1473.2)
  line L13 (12.7, -1473.2) -> (228.6, -1473.2)
  line L14 (228.6, -1473.2) -> (228.6, -1676.4)
  line L15 (228.6, -1676.4) -> (12.7, -1676.4)
  line L16 (-165.1, -203.2) -> (-254, -203.2)
  line L17 (-254, -203.2) -> (-254, -25.4)
  line L18 (-254, -25.4) -> (-165.1, -25.4)
  line L19 (-165.1, -25.4) -> (-165.1, -203.2)
  line L20 (-355.6, -228.6) -> (-279.4, -228.6)
  line L21 (-279.4, -228.6) -> (-279.4, -355.6)
  line L22 (-279.4, -355.6) -> (-355.6, -355.6)
  line L23 (-355.6, -355.6) -> (-355.6, -228.6)
  line L24 (-12.7, -711.2) -> (-12.7, -1447.8)
  line L25 (-12.7, -1447.8) -> (-228.6, -1447.8)
  line L26 (-228.6, -1447.8) -> (-228.6, -1446.1784)
  line L27 (-228.6, -1446.1784) -> (-322.828, -711.2)
  line L28 (-322.828, -711.2) -> (-12.7, -711.2)
  line L29 (-139.7, -203.2) -> (-139.7, -25.4)
  line L30 (-139.7, -25.4) -> (355.6, -25.4)
  line L31 (355.6, -25.4) -> (355.6, -203.2)
  line L32 (355.6, -203.2) -> (-139.7, -203.2)
  line L33 (228.6, -1701.8) -> (228.6, -1879.6)
  line L34 (228.6, -1879.6) -> (12.7, -1879.6)
  line L35 (12.7, -1879.6) -> (12.7, -1701.8)
  line L36 (12.7, -1701.8) -> (228.6, -1701.8)
  line L37 (-355.6, -455.5784) -> (-355.3921, -457.2)
  line L38 (-355.3921, -457.2) -> (-12.7, -457.2)
  line L39 (-12.7, -457.2) -> (-12.7, -685.8)
  line L40 (-12.7, -685.8) -> (-326.0844, -685.8)
  line L41 (-326.0844, -685.8) -> (-355.3921, -457.2)
  line L42 (-355.3921, -457.2) -> (-355.6, -457.2)
  line L43 (-355.6, -457.2) -> (-355.6, -455.5784)
  line L44 (-12.7, -1676.4) -> (-228.6, -1676.4)
  line L45 (-228.6, -1676.4) -> (-228.6, -1473.2)
  line L46 (-228.6, -1473.2) -> (-12.7, -1473.2)
  line L47 (-12.7, -1473.2) -> (-12.7, -1676.4)
  line L48 (-165.1, -355.6) -> (-254, -355.6)
  line L49 (-254, -355.6) -> (-254, -228.6)
  line L50 (-254, -228.6) -> (-165.1, -228.6)
  line L51 (-165.1, -228.6) -> (-165.1, -355.6)
  line L52 (-355.6, -381) -> (355.6, -381)
  line L53 (355.6, -381) -> (355.6, -431.8)
  line L54 (355.6, -431.8) -> (-355.6, -431.8)
  line L55 (-355.6, -431.8) -> (-355.6, -381)
  line L56 (12.7, -685.8) -> (12.7, -457.2)
  line L57 (12.7, -457.2) -> (355.3921, -457.2)
  line L58 (355.3921, -457.2) -> (355.6, -455.5784)
  line L59 (355.6, -455.5784) -> (355.6, -457.2)
  line L60 (355.6, -457.2) -> (355.3921, -457.2)
  line L61 (355.3921, -457.2) -> (326.0844, -685.8)
  line L62 (326.0844, -685.8) -> (12.7, -685.8)
  line L63 (-139.7, -228.6) -> (355.6, -228.6)
  line L64 (355.6, -228.6) -> (355.6, -355.6)
  line L65 (355.6, -355.6) -> (-139.7, -355.6)
  line L66 (-139.7, -355.6) -> (-139.7, -228.6)
  line L67 (228.6, -1446.1784) -> (228.6, -1447.8)
  line L68 (228.6, -1447.8) -> (12.7, -1447.8)
  line L69 (12.7, -1447.8) -> (12.7, -711.2)
  line L70 (12.7, -711.2) -> (322.828, -711.2)
  line L71 (322.828, -711.2) -> (228.6, -1446.1784)
  line L72 (-273.5385, -1295.4) -> (-498.8821, -1295.4)
  line L73 (-498.8821, -1295.4) -> (-498.8821, -711.2)
  line L74 (-498.8821, -711.2) -> (-348.4359, -711.2)
  line L75 (-348.4359, -711.2) -> (-273.5385, -1295.4)
  line L76 (270.2821, -1320.8) -> (524.2821, -1320.8)
  line L77 (524.2821, -1320.8) -> (524.2821, -685.8)
  line L78 (524.2821, -685.8) -> (351.6923, -685.8)
  line L79 (351.6923, -685.8) -> (381, -457.2)
  line L80 (381, -457.2) -> (381, -228.6)
  line L81 (381, -228.6) -> (393.7, -228.6)
  line L82 (393.7, -228.6) -> (393.7, -203.2)
  line L83 (393.7, -203.2) -> (381, -203.2)
  line L84 (381, -203.2) -> (381, 0)
  line L85 (381, 0) -> (-381, 0)
  line L86 (-381, 0) -> (-381, -203.2)
  line L87 (-381, -203.2) -> (-508, -203.2)
  line L88 (-508, -203.2) -> (-508, -228.6)
  line L89 (-508, -228.6) -> (-381, -228.6)
  line L90 (-381, -228.6) -> (-381, -457.2)
  line L91 (-381, -457.2) -> (-351.6923, -685.8)
  line L92 (-351.6923, -685.8) -> (-524.2821, -685.8)
  line L93 (-524.2821, -685.8) -> (-524.2821, -1320.8)
  line L94 (-524.2821, -1320.8) -> (-270.2821, -1320.8)
  line L95 (-270.2821, -1320.8) -> (-254, -1447.8)
  line L96 (-254, -1447.8) -> (-254, -1676.4)
  line L97 (-254, -1676.4) -> (-393.7, -1676.4)
  line L98 (-393.7, -1676.4) -> (-393.7, -1701.8)
  line L99 (-393.7, -1701.8) -> (-254, -1701.8)
  line L100 (-254, -1701.8) -> (-254, -1905)
  line L101 (-254, -1905) -> (254, -1905)
  line L102 (254, -1905) -> (254, -1701.8)
  line L103 (254, -1701.8) -> (393.7, -1701.8)
  line L104 (393.7, -1701.8) -> (393.7, -1676.4)
  line L105 (393.7, -1676.4) -> (254, -1676.4)
  line L106 (254, -1676.4) -> (254, -1447.8)
  line L107 (254, -1447.8) -> (270.2821, -1320.8)
  line L108 (-184.15, -482.6) -> (184.15, -482.6)
  line L109 (184.15, -482.6) -> (184.15, -800.1)
  line L110 (-184.15, -482.6) -> (-184.15, -800.1)
  arc A0 (184.15, -800.1) -> (-184.15, -800.1) centre (0, -1086.689) ccw
  circle A1 centre (158.75, -698.5) radius 3
  circle A2 centre (-158.75, -698.5) radius 3
  circle A3 centre (0, -508) radius 3
  circle A4 centre (-158.75, -698.5) radius 4
  circle A5 centre (158.75, -698.5) radius 4
  circle A6 centre (0, -508) radius 4
  point P0 (0, -482.6)
  point P1 (0, -482.6)
  dimension "d325" = 368.3
  dimension "d326" = 317.5
  dimension "d327" = 317.5
  dimension "d330" = 6
  dimension "d331" = 12.7
  dimension "d332" = 25.4
  dimension "d333" = 6
  dimension "d334" = 25.4
  dimension "d335" = 12.7
  dimension "d336" = 6
  dimension "d337" = 25.4
  dimension "d338" = 12.7
  dimension "d339" = 8
  dimension "d340" = 8
  dimension "d341" = 8
  constraint midpoint L108 P1
  constraint coincident P1 P0
  constraint perpendicular L39 L108
  constraint perpendicular L70 L109
  constraint perpendicular L108 L110
  constraint concentric A2 A4
  constraint concentric A1 A5
  constraint concentric A3 A6
  measures "d325" distance of L108.start L108.end
  measures "d326" distance of L108.end L109.end
  measures "d327" distance of L108.start L110.end
  measures "d330" diameter of A1
  measures "d331" distance of L70 A1.centre
  measures "d332" distance of L109 A1.centre
  measures "d333" diameter of A2
  measures "d334" distance of L110 A2.centre
  measures "d335" distance of L40 A2.centre
  measures "d336" diameter of A3
  measures "d337" vertical distance of P1 A3.centre
  measures "d338" distance of L56 A3.centre
  measures "d339" diameter of A4
  measures "d340" diameter of A5
  measures "d341" diameter of A6
extrude "Extrude25" add sketch "Sketch22" along normal blind 12.7 separate body contours L24 L28 L39 L40 L56 L62 L69 L70 L108 L109 L110 A0 | L24 L28 L110 A0 | L69 L70 L109 A0 | L39 L40 L108 L110 | L56 L62 L108 L109 | A4 | A5 | A6 makes body 22
extrude "Extrude26" add sketch "Sketch22" along normal blind 16.7 separate body contours A1 | A2 | A3 | A4 | A5 | A6 makes body 23 at (-3.8763, 507.013, 36.5333) makes body 24 at (154.8737, 697.513, 36.5333) makes body 25 at (-162.6263, 697.513, 36.5333)
chamfer "Chamfer1" distance 2 angle 45 3 edges at (-155.0207, 699.9465, 42.1) (3.7293, 509.4465, 42.1) (162.4793, 699.9465, 42.1) on bodies 23 24 25